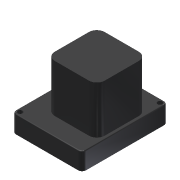
# Autodesk Inventor part: Victor Controller
Saved by Autodesk Inventor 2013 (Build 170138000, 138)
## iProperties
Created: 2013-12-22
Part Number: Victor Controller
Material: Nylon 6/6
Document SubType Name: Modeling
Designer: Nemo
Density: 1.00523 g/cm^3
Mass: 113.398 g
Surface Area: 169.534 cm^2
Volume: 112.809 cm^3
Author: Nemo
Autodesk Inventor part; units mm, degrees
ref_plane "YZ Plane" through (0, 0, 0) normal (1, 0, 0) x (0, 1, 0)
ref_plane "XZ Plane" through (0, 0, 0) normal (0, 1, 0) x (-1, 0, 0)
ref_plane "XY Plane" through (0, 0, 0) normal (0, 0, 1) x (1, 0, 0)
sketch "Sketch2" plane through (0, 0, 0) normal (0, 1, 0) x (-1, 0, 0)
  circle A0 centre (49.6189, -7.9375) radius 2.6988 construction
  circle A1 centre (0, -3.175) radius 2.6988 construction
  circle A2 centre (49.6189, -3.175) radius 1.905
  circle A3 centre (0, -65.405) radius 1.905
  arc A4 (49.6189, -68.58) -> (52.7939, -65.405) centre (49.6189, -65.405) ccw
  line L0 (52.7939, -65.405) -> (52.7939, -3.175)
  arc A5 (52.7939, -3.175) -> (49.6189, 0) centre (49.6189, -3.175) ccw
  line L1 (49.6189, 0) -> (0, 0)
  arc A6 (0, 0) -> (-3.175, -3.175) centre (0, -3.175) ccw
  line L2 (-3.175, -3.175) -> (-3.175, -65.405)
  arc A7 (-3.175, -65.405) -> (0, -68.58) centre (0, -65.405) ccw
  line L3 (0, -68.58) -> (49.6189, -68.58)
  circle A8 centre (49.6189, -65.405) radius 2.6988 construction
  circle A9 centre (0, -60.6425) radius 2.6988 construction
  point P0 (24.8095, -34.29)
  constraints: 10 centre point, 8 end point, 8 point on circle
extrude "Extrusion1" add sketch "Sketch2" along normal blind 13.97
fillet "Fillet1" radius 0.762 8 edges at (-52.7939, 13.97, -34.29) (-51.864, 13.97, -0.9299) (-24.8095, 13.97, 0) (2.2451, 13.97, -0.9299) (3.175, 13.97, -34.29) (2.2451, 13.97, -67.6501) (-24.8095, 13.97, -68.58) (-51.864, 13.97, -67.6501)
sketch "Sketch3" plane through (0, 13.97, 0) normal (0, 1, 0) x (1, 0, 0)
  line L0 (-52.0319, 3.175) -> (-52.0319, 65.405) projected
  line L1 (-39.37, 54.2925) -> (0.635, 54.2925)
  line L2 (0.635, 54.2925) -> (0.635, 14.2875)
  line L3 (0.635, 14.2875) -> (-39.37, 14.2875)
  line L4 (-39.37, 14.2875) -> (-39.37, 54.2925)
  line L5 (3.175, 3.175) -> (3.175, 65.405) projected
  point P0 (0, 0)
  point P1 (-52.0319, 34.29)
  point P2 (-39.37, 34.29)
  dimension "d3" = 40.005
  dimension "d4" = 40.005
  dimension "d5" = 2.54
  constraints: 8 end point, 2 midpoint, 2 parallel, 1 horizontal, 1 horizontal alignment, 1 perpendicular
  measures "d3" distance of L2.end L3.end
  measures "d4" distance of L1.end L2.end
  measures "d5" distance between parallel lines of L5 L2
extrude "Extrusion2" add sketch "Sketch3" along normal blind 38.1
fillet "Fillet2" radius 6.35 4 edges at (-39.37, 33.02, -14.2875) (0.635, 33.02, -14.2875) (0.635, 33.02, -54.2925) (-39.37, 33.02, -54.2925)
body "Solid1"
